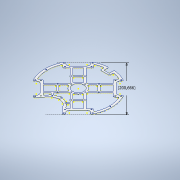
# Autodesk Inventor part: upper_plate_04
Saved by Autodesk Inventor 2020 (Build 240168000, 168)
## iProperties
Created: 2023-12-20
Part Number: upper_plate_04
Material: Алюминий 6061
Document SubType Name: Modeling
Designer: denis
Density: 2.71714 g/cm^3
Appearance: Алюминий — плоский
Mass: 51 g
Surface Area: 248.649 cm^2
Volume: 18.7698 cm^3
Author: denis
Autodesk Inventor part; units mm, degrees
(part 1 of 3)
ref_plane "YZ Plane" through (0, 0, 0) normal (1, 0, 0) x (0, 1, 0)
ref_plane "XZ Plane" through (0, 0, 0) normal (0, 1, 0) x (-1, 0, 0)
ref_plane "XY Plane" through (0, 0, 0) normal (0, 0, 1) x (1, 0, 0)
sketch "Эскиз1" plane through (0, 0, 0) normal (0, 1, 0) x (-1, 0, 0)
  arc A0 (93.0503, -48.6481) -> (93.0503, 48.6481) centre (0, 0) ccw
  line L0 (0, 0) -> (0, -105) construction
  line L1 (0, 0) -> (105, 0) construction
  line L2 (0, 0) -> (74.2462, -74.2462) construction
  line L3 (0, 0) -> (105, 0) construction
  arc A1 (47.0668, -85.9577) -> (85.9577, -47.0668) centre (0, 0) ccw construction
  line L4 (0, 0) -> (-74.2462, -74.2462) construction
  line L5 (73.8927, -46.3155) -> (46.3155, -73.8927)
  line L6 (76.014, -34.2947) -> (34.2947, -76.014)
  circle A2 centre (37.8302, -79.5495) radius 1.6
  circle A3 centre (79.5495, -37.8302) radius 1.6
  line L7 (37.8302, -79.5495) -> (79.5495, -37.8302) construction
  line L8 (87.1795, -38.3892) -> (83.085, -34.2947)
  line L9 (38.3892, -87.1795) -> (34.2947, -83.085)
  line L10 (88.2704, -49.3795) -> (85.2064, -46.3155)
  line L11 (49.3795, -88.2704) -> (46.3155, -85.2064)
  arc A4 (74.2462, -74.2462) -> (91.1, -52.2091) centre (0, 0) ccw construction
  arc A5 (52.2091, -91.1) -> (74.2462, -74.2462) centre (0, 0) ccw construction
  arc A6 (48.6481, -93.0503) -> (49.3795, -88.2704) centre (47.2582, -90.3917) ccw
  arc A7 (88.2704, -49.3795) -> (93.0503, -48.6481) centre (90.3917, -47.2582) ccw
  arc A8 (46.3155, -73.8927) -> (46.3155, -85.2064) centre (51.9723, -79.5495) ccw
  arc A9 (85.2064, -46.3155) -> (73.8927, -46.3155) centre (79.5495, -51.9723) ccw
  arc A10 (34.2947, -76.014) -> (34.2947, -83.085) centre (37.8302, -79.5495) ccw
  arc A11 (83.085, -34.2947) -> (76.014, -34.2947) centre (79.5495, -37.8302) ccw
  arc A12 (40.4652, -89.2556) -> (47.0668, -85.9577) centre (0, 0) ccw construction
  arc A13 (85.9577, -47.0668) -> (89.2556, -40.4652) centre (0, 0) ccw construction
  arc A14 (90.4395, -37.7453) -> (90.4395, 37.7453) centre (0, 0) ccw
  arc A15 (87.1795, -38.3892) -> (90.4395, -37.7453) centre (88.5938, -36.975) ccw
  arc A16 (37.7453, -90.4395) -> (38.3892, -87.1795) centre (36.975, -88.5938) ccw
  arc A17 (38.3892, 87.1795) -> (37.7453, 90.4395) centre (36.975, 88.5938) ccw construction
  arc A18 (49.3795, 88.2704) -> (48.6481, 93.0503) centre (47.2582, 90.3917) ccw
  line L12 (49.3795, 88.2704) -> (46.3155, 85.2064)
  arc A19 (46.3155, 85.2064) -> (46.3155, 73.8927) centre (51.9723, 79.5495) ccw
  line L13 (38.3892, 87.1795) -> (34.2947, 83.085) construction
  arc A20 (34.2947, 83.085) -> (34.2947, 76.014) centre (37.8302, 79.5495) ccw construction
  line L14 (34.2947, 76.014) -> (76.014, 34.2947) construction
  line L15 (46.3155, 73.8927) -> (73.8927, 46.3155)
  arc A21 (76.014, 34.2947) -> (83.085, 34.2947) centre (79.5495, 37.8302) ccw
  circle A22 centre (37.8302, 79.5495) radius 1.6
  circle A23 centre (79.5495, 37.8302) radius 1.6
  line L16 (87.1795, 38.3892) -> (83.085, 34.2947)
  arc A24 (90.4395, 37.7453) -> (87.1795, 38.3892) centre (88.5938, 36.975) ccw
  arc A25 (93.0503, 48.6481) -> (88.2704, 49.3795) centre (90.3917, 47.2582) ccw
  line L17 (88.2704, 49.3795) -> (85.2064, 46.3155)
  arc A26 (73.8927, 46.3155) -> (85.2064, 46.3155) centre (79.5495, 51.9723) ccw
  arc A27 (-87.1795, 38.3892) -> (-90.4395, 37.7453) centre (-88.5938, 36.975) ccw
  arc A28 (-88.2704, 49.3795) -> (-93.0503, 48.6481) centre (-90.3917, 47.2582) ccw
  line L18 (-88.2704, 49.3795) -> (-85.2064, 46.3155)
  arc A29 (-85.2064, 46.3155) -> (-73.8927, 46.3155) centre (-79.5495, 51.9723) ccw
  line L19 (-87.1795, 38.3892) -> (-83.085, 34.2947)
  arc A30 (-83.085, 34.2947) -> (-76.014, 34.2947) centre (-79.5495, 37.8302) ccw
  line L20 (-76.014, 34.2947) -> (-34.2947, 76.014) construction
  line L21 (-73.8927, 46.3155) -> (-46.3155, 73.8927)
  arc A31 (-34.2947, 76.014) -> (-34.2947, 83.085) centre (-37.8302, 79.5495) ccw construction
  circle A32 centre (-79.5495, 37.8302) radius 1.6
  circle A33 centre (-37.8302, 79.5495) radius 1.6
  line L22 (-38.3892, 87.1795) -> (-34.2947, 83.085) construction
  arc A34 (-37.7453, 90.4395) -> (-38.3892, 87.1795) centre (-36.975, 88.5938) ccw construction
  arc A35 (-48.6481, 93.0503) -> (-49.3795, 88.2704) centre (-47.2582, 90.3917) ccw
  line L23 (-49.3795, 88.2704) -> (-46.3155, 85.2064)
  arc A36 (-46.3155, 73.8927) -> (-46.3155, 85.2064) centre (-51.9723, 79.5495) ccw
  arc A37 (-38.3892, -87.1795) -> (-37.7453, -90.4395) centre (-36.975, -88.5938) ccw
  arc A38 (-49.3795, -88.2704) -> (-48.6481, -93.0503) centre (-47.2582, -90.3917) ccw
  line L24 (-49.3795, -88.2704) -> (-46.3155, -85.2064)
  arc A39 (-46.3155, -85.2064) -> (-46.3155, -73.8927) centre (-51.9723, -79.5495) ccw
  line L25 (-38.3892, -87.1795) -> (-34.2947, -83.085)
  arc A40 (-34.2947, -83.085) -> (-34.2947, -76.014) centre (-37.8302, -79.5495) ccw
  line L26 (-34.2947, -76.014) -> (-76.014, -34.2947)
  line L27 (-46.3155, -73.8927) -> (-73.8927, -46.3155)
  arc A41 (-76.014, -34.2947) -> (-83.085, -34.2947) centre (-79.5495, -37.8302) ccw
  circle A42 centre (-37.8302, -79.5495) radius 1.6
  circle A43 centre (-79.5495, -37.8302) radius 1.6
  line L28 (-87.1795, -38.3892) -> (-83.085, -34.2947)
  arc A44 (-90.4395, -37.7453) -> (-87.1795, -38.3892) centre (-88.5938, -36.975) ccw
  arc A45 (-93.0503, -48.6481) -> (-88.2704, -49.3795) centre (-90.3917, -47.2582) ccw
  line L29 (-88.2704, -49.3795) -> (-85.2064, -46.3155)
  arc A46 (-73.8927, -46.3155) -> (-85.2064, -46.3155) centre (-79.5495, -51.9723) ccw
  arc A47 (0, 67.941) -> (23.7825, 76.5969) centre (0, 104.941) ccw construction
  arc A48 (-23.7825, 76.5969) -> (0, 67.941) centre (0, 104.941) ccw construction
  line L30 (-23.7825, 76.5969) -> (-29.1816, 81.127) construction
  arc A49 (-28.5452, 71.4571) -> (5.5413, 61.2914) centre (0, 104.941) ccw construction
  arc A50 (5.5413, 61.2914) -> (28.5452, 71.4571) centre (0, 104.941) ccw construction
  line L31 (23.7825, 76.5969) -> (26.8032, 79.1314) construction
  line L32 (-34.1491, 76.1596) -> (-28.5452, 71.4571) construction
  line L33 (31.2232, 73.7044) -> (28.5452, 71.4571) construction
  line L34 (26.8032, 79.1314) -> (23.7825, 76.5969) construction
  line L35 (30.7591, 79.5495) -> (31.4483, 78.8604) construction
  line L36 (31.2232, 73.7044) -> (28.5452, 71.4571) construction
  line L37 (-28.5452, 71.4571) -> (-34.1491, 76.1596) construction
  line L38 (-23.7825, 76.5969) -> (-29.1816, 81.127) construction
  line L39 (-29.1816, 81.127) -> (-34.1491, 76.1596) construction
  arc A51 (31.2232, 73.7044) -> (26.6462, 78.9996) centre (28.9734, 76.3855) ccw construction
  arc A52 (-26.6462, 78.9996) -> (-31.2232, 73.7044) centre (-28.9734, 76.3855) ccw construction
  arc A53 (-24.842, 61.8893) -> (-25.4187, 62.8242) centre (-28.1154, 60.5155) ccw
  line L40 (-24.842, 61.8893) -> (-23.8313, 59.4808)
  line L41 (-43.0355, 94.1655) -> (-18.3802, 65.3664)
  arc A54 (-0.6161, 59.3045) -> (0.6161, 59.3045) centre (0, 61.2072) ccw
  line L42 (-2.672, 59.9702) -> (-4.5, 60.5621) construction
  arc A55 (-2.5156, 60.0805) -> (-2.672, 59.9702) centre (0, 56.3493) ccw construction
  line L43 (-15.1585, 56.5907) -> (-21.0049, 57.3328)
  arc A56 (-14.5119, 56.4463) -> (-15.1585, 56.5907) centre (-15.6055, 53.069) ccw
  line L44 (-17.477, 64.7643) -> (-0.6161, 59.3045)
  line L45 (-14.5119, 56.4463) -> (-0.6161, 51.9466)
  arc A57 (44.0271, 95.3237) -> (43.577, 95.5303) centre (0, 0) ccw construction
  circle A58 centre (20.5578, 60.8546) radius 1.55
  arc A59 (-34.1909, 73.0707) -> (-37.1244, 73.1843) centre (-35.7102, 71.7701) ccw
  line L46 (-34.1909, 73.0707) -> (-27.0558, 64.7365) construction
  line L47 (-25.4187, 62.8242) -> (-34.1909, 73.0707)
  arc A60 (-23.8313, 59.4808) -> (-21.0049, 57.3328) centre (-20.5578, 60.8546) ccw
  arc A61 (-18.3802, 65.3664) -> (-17.477, 64.7643) centre (-16.8609, 66.6671) ccw
  circle A62 centre (-20.5578, 60.8546) radius 1.55
  arc A63 (15.1585, 56.5907) -> (14.5119, 56.4463) centre (15.6055, 53.069) ccw
  line L48 (15.1585, 56.5907) -> (21.0049, 57.3328)
  arc A64 (25.4187, 62.8242) -> (24.842, 61.8893) centre (28.1154, 60.5155) ccw
  line L49 (24.842, 61.8893) -> (23.8313, 59.4808)
  arc A65 (21.0049, 57.3328) -> (23.8313, 59.4808) centre (20.5578, 60.8546) ccw
  line L50 (25.4187, 62.8242) -> (34.1909, 73.0707)
  arc A66 (37.1244, 73.1843) -> (34.1909, 73.0707) centre (35.7102, 71.7701) ccw
  line L51 (14.5119, 56.4463) -> (0.6161, 51.9466)
  arc A67 (17.477, 64.7643) -> (18.3802, 65.3664) centre (16.8609, 66.6671) ccw
  line L52 (17.477, 64.7643) -> (0.6161, 59.3045)
  line L53 (-37.1244, 73.1843) -> (-76.014, 34.2947)
  line L54 (37.1244, 73.1843) -> (76.014, 34.2947)
  arc A68 (-45.42, 94.668) -> (-48.6481, 93.0503) centre (0, 0) ccw
  arc A69 (-43.0355, 94.1655) -> (-45.42, 94.668) centre (-44.5548, 92.8648) ccw
  arc A70 (-0.6161, 51.9466) -> (0.6161, 51.9466) centre (0, 53.8493) ccw
  arc A71 (-48.6481, 93.0503) -> (-93.0503, 48.6481) centre (0, 0) ccw construction
  line L55 (43.0355, 94.1655) -> (18.3802, 65.3664)
  arc A72 (48.6481, 93.0503) -> (45.42, 94.668) centre (0, 0) ccw
  arc A73 (45.42, 94.668) -> (43.0355, 94.1655) centre (44.5548, 92.8648) ccw
  arc A74 (93.0503, 48.6481) -> (-44.0271, 95.3237) centre (0, 0) ccw construction
  arc A75 (-93.0503, -48.6481) -> (-48.6481, -93.0503) centre (0, 0) ccw construction
  arc A76 (-93.0503, 48.6481) -> (-93.0503, -48.6481) centre (0, 0) ccw
  arc A77 (-90.4395, -37.7453) -> (-37.7453, -90.4395) centre (0, 0) ccw construction
  arc A78 (-90.4395, 37.7453) -> (-90.4395, -37.7453) centre (0, 0) ccw
  arc A79 (90.4395, 37.7453) -> (-90.4395, 37.7453) centre (0, 0) ccw construction
  arc A80 (-37.7453, -90.4395) -> (37.7453, -90.4395) centre (0, 0) ccw
  arc A81 (-48.6481, -93.0503) -> (48.6481, -93.0503) centre (0, 0) ccw
  circle A82 centre (0, 55.4493) radius 1.6
  point P0 (60.1041, -60.1041)
  point P1 (55.1543, -55.1543)
  point P2 (78.1353, -39.2444)
  point P3 (39.2444, -78.1353)
  point P4 (52.2091, 91.1)
  point P5 (39.2444, 78.1353)
  point P6 (47.0668, 85.9577)
  point P7 (55.1543, 55.1543)
  point P8 (60.1041, 60.1041)
  point P9 (91.1, 52.2091)
  point P10 (78.1353, 39.2444)
  point P11 (85.9577, 47.0668)
  point P12 (-91.1, 52.2091)
  point P13 (-78.1353, 39.2444)
  point P14 (-85.9577, 47.0668)
  point P15 (-55.1543, 55.1543)
  point P16 (-60.1041, 60.1041)
  point P17 (-52.2091, 91.1)
  point P18 (-39.2444, 78.1353)
  point P19 (-47.0668, 85.9577)
  point P20 (-52.2091, -91.1)
  point P21 (-39.2444, -78.1353)
  point P22 (-47.0668, -85.9577)
  point P23 (-55.1543, -55.1543)
  point P24 (-60.1041, -60.1041)
  point P25 (-91.1, -52.2091)
  point P26 (-78.1353, -39.2444)
  point P27 (-85.9577, -47.0668)
  point P28 (-28.5452, 71.4571)
  point P29 (-39.283, 89.7822)
  point P30 (0, 95.3237)
  point P31 (0, 66.2072)
  point P32 (-44.0271, 95.3237)
  point P33 (0, 59.2072)
  point P34 (44.5548, 92.8648)
  point P35 (-42.4264, 67.8823)
  point P36 (-22.7059, 58.0282)
  point P37 (-21.4957, 59.6205)
  dimension "d1" = 45
  dimension "d3" = 7
  dimension "d5" = 20
  dimension "d9" = 7
  dimension "d10" = 3.2
  dimension "d14" = 59
  dimension "d15" = 83
  dimension "d17" = 69
  dimension "d19" = 55
  dimension "d20" = 3
  dimension "d21" = 8
  dimension "d22" = 5
  dimension "d23" = 2
  dimension "d26" = 360
  dimension "d39" = 7
  dimension "d44" = 120
  dimension "d45" = 3.55
  dimension "d46" = 2
  dimension "d47" = 2.6119
  dimension "d48" = 2
  dimension "d49" = 105
  dimension "d50" = 2
  dimension "d54" = 3.2
  dimension "d55" = 2
  constraints: 165 point on circle, 112 end point, 83 centre point, 38 point on line, 27 tangent, 23 symmetric about line, 8 midpoint, 6 equal radius, 4 coincident, 4 collinear, 4 parallel, 3 horizontal, 2 vertical, 1 equal length, 1 perpendicular, 234 other
  measures "d1" angle of L2 L3
  measures "d3" radial gap between concentric circles of A0 A1
  measures "d5" distance from line of L5 L2.end
  measures "d9" distance between parallel lines of L5 L6
  measures "d10" diameter of A2
  measures "d14" distance of L7.end L7.start
  measures "d15" distance from line of point (0, 0) L7
  measures "d17" distance between parallel lines of L8 L9
  measures "d19" distance between parallel lines of L11 L10
  measures "d20" radius of A6
  measures "d21" radius of A8
  measures "d22" radius of A10
  measures "d23" radius of A15
  measures "d39" distance of point (0, 66.207) point (0, 59.207)
  measures "d44" angle of L40 L43
  measures "d45" radius of A53
  measures "d46" distance of point (-22.706, 58.028) point (-21.496, 59.621)
  measures "d47" distance of L40.start L40.end
  measures "d48" radius of A69
  measures "d49" radius of A68
  measures "d50" radius of A70
  measures "d54" diameter of A82
extrude "outer" add sketch "Эскиз1" along normal blind 2 contours A7 L10 A9 L5 A8 L11 A6 A81 A38 L24 A39 L27 A46 L29 A45 A76 A28 L18 A29 L21 A36 L23 A35 A68 A69 L41 A61 L44 A54 L52 A67 L55 A73 A72 A18 L12 A19 L15 A26 L17 A25 A0 | A82
sketch "Эскиз2" plane through (0, 2, 0) normal (0, 1, 0) x (1, 0, 0)
  circle A0 centre (0, 0) radius 18
  arc A1 (-16.2635, 16.2635) -> (-21.4111, 8.4003) centre (0, 0) ccw
  line L0 (0, 0) -> (-74.2462, 74.2462) construction
  line L1 (0, 0) -> (-105, 0) construction
  line L2 (0, 0) -> (0, 105) construction
  line L3 (0, 0) -> (74.2462, 74.2462) construction
  line L4 (-46.669, 63.6396) -> (-27.2236, 44.1942)
  line L5 (-63.6396, 46.669) -> (-44.1942, 27.2236)
  arc A2 (-46.3155, -85.2064) -> (-46.3155, -73.8927) centre (-51.9723, -79.5495) ccw construction
  line L6 (-46.3155, -85.2064) -> (-49.3795, -88.2704) construction
  arc A3 (-49.3795, -88.2704) -> (-48.6481, -93.0503) centre (-47.2582, -90.3917) ccw construction
  arc A4 (-48.6481, -93.0503) -> (-45.42, -94.668) centre (0, 0) ccw construction
  arc A5 (-45.42, -94.668) -> (-43.0355, -94.1655) centre (-44.5548, -92.8648) ccw construction
  line L7 (-43.0355, -94.1655) -> (-18.3802, -65.3664) construction
  arc A6 (-17.477, -64.7643) -> (-18.3802, -65.3664) centre (-16.8609, -66.6671) ccw construction
  line L8 (-17.477, -64.7643) -> (-0.6161, -59.3045) construction
  arc A7 (0.6161, -59.3045) -> (-0.6161, -59.3045) centre (0, -61.2072) ccw construction
  line L9 (0.6161, -59.3045) -> (17.477, -64.7643) construction
  arc A8 (18.3802, -65.3664) -> (17.477, -64.7643) centre (16.8609, -66.6671) ccw construction
  line L10 (18.3802, -65.3664) -> (43.0355, -94.1655) construction
  arc A9 (43.0355, -94.1655) -> (45.42, -94.668) centre (44.5548, -92.8648) ccw construction
  arc A10 (45.42, -94.668) -> (48.6481, -93.0503) centre (0, 0) ccw construction
  arc A11 (48.6481, -93.0503) -> (49.3795, -88.2704) centre (47.2582, -90.3917) ccw construction
  line L11 (49.3795, -88.2704) -> (46.3155, -85.2064) construction
  arc A12 (46.3155, -73.8927) -> (46.3155, -85.2064) centre (51.9723, -79.5495) ccw construction
  line L12 (46.3155, -73.8927) -> (73.8927, -46.3155) construction
  arc A13 (85.2064, -46.3155) -> (73.8927, -46.3155) centre (79.5495, -51.9723) ccw construction
  line L13 (85.2064, -46.3155) -> (88.2704, -49.3795) construction
  arc A14 (88.2704, -49.3795) -> (93.0503, -48.6481) centre (90.3917, -47.2582) ccw construction
  arc A15 (93.0503, -48.6481) -> (93.0503, 48.6481) centre (0, 0) ccw construction
  arc A16 (93.0503, 48.6481) -> (88.2704, 49.3795) centre (90.3917, 47.2582) ccw construction
  line L14 (88.2704, 49.3795) -> (85.2064, 46.3155) construction
  arc A17 (73.8927, 46.3155) -> (85.2064, 46.3155) centre (79.5495, 51.9723) ccw construction
  line L15 (73.8927, 46.3155) -> (46.3155, 73.8927) construction
  arc A18 (46.3155, 85.2064) -> (46.3155, 73.8927) centre (51.9723, 79.5495) ccw construction
  line L16 (46.3155, 85.2064) -> (49.3795, 88.2704) construction
  arc A19 (49.3795, 88.2704) -> (48.6481, 93.0503) centre (47.2582, 90.3917) ccw construction
  arc A20 (48.6481, 93.0503) -> (-48.6481, 93.0503) centre (0, 0) ccw construction
  arc A21 (-48.6481, 93.0503) -> (-49.3795, 88.2704) centre (-47.2582, 90.3917) ccw construction
  line L17 (-49.3795, 88.2704) -> (-46.3155, 85.2064) construction
  arc A22 (-46.3155, 73.8927) -> (-46.3155, 85.2064) centre (-51.9723, 79.5495) ccw construction
  line L18 (-46.3155, 73.8927) -> (-73.8927, 46.3155) construction
  arc A23 (-85.2064, 46.3155) -> (-73.8927, 46.3155) centre (-79.5495, 51.9723) ccw construction
  line L19 (-85.2064, 46.3155) -> (-88.2704, 49.3795) construction
  arc A24 (-88.2704, 49.3795) -> (-93.0503, 48.6481) centre (-90.3917, 47.2582) ccw construction
  arc A25 (-93.0503, 48.6481) -> (-93.0503, -48.6481) centre (0, 0) ccw construction
  arc A26 (-93.0503, -48.6481) -> (-88.2704, -49.3795) centre (-90.3917, -47.2582) ccw construction
  line L20 (-88.2704, -49.3795) -> (-85.2064, -46.3155) construction
  arc A27 (-73.8927, -46.3155) -> (-85.2064, -46.3155) centre (-79.5495, -51.9723) ccw construction
  line L21 (-73.8927, -46.3155) -> (-46.3155, -73.8927) construction
  circle A28 centre (-37.8302, 79.5495) radius 1.6 construction
  circle A29 centre (-79.5495, 37.8302) radius 1.6 construction
  circle A30 centre (-79.5495, -37.8302) radius 1.6 construction
  circle A31 centre (79.5495, -37.8302) radius 1.6 construction
  circle A32 centre (37.8302, 79.5495) radius 1.6 construction
  circle A33 centre (79.5495, 37.8302) radius 1.6 construction
  circle A34 centre (-20.5578, -60.8546) radius 1.55 construction
  circle A35 centre (20.5578, -60.8546) radius 1.55 construction
  circle A36 centre (37.8302, -79.5495) radius 1.6 construction
  circle A37 centre (-37.8302, -79.5495) radius 1.6 construction
  line L22 (-83.085, -34.2947) -> (-87.1795, -38.3892) construction
  arc A38 (-90.4395, -37.7453) -> (-87.1795, -38.3892) centre (-88.5938, -36.975) ccw construction
  arc A39 (-90.4395, 37.7453) -> (-90.4395, -37.7453) centre (0, 0) ccw construction
  arc A40 (-87.1795, 38.3892) -> (-90.4395, 37.7453) centre (-88.5938, 36.975) ccw construction
  line L23 (-87.1795, 38.3892) -> (-83.085, 34.2947) construction
  arc A41 (-83.085, 34.2947) -> (-76.014, 34.2947) centre (-79.5495, 37.8302) ccw construction
  line L24 (-76.014, 34.2947) -> (-34.2947, 76.014) projected
  arc A42 (-34.2947, 76.014) -> (-34.2947, 83.085) centre (-37.8302, 79.5495) ccw construction
  line L25 (-34.2947, 83.085) -> (-38.3892, 87.1795) construction
  arc A43 (-37.7453, 90.4395) -> (-38.3892, 87.1795) centre (-36.975, 88.5938) ccw construction
  arc A44 (37.7453, 90.4395) -> (-37.7453, 90.4395) centre (0, 0) ccw construction
  arc A45 (38.3892, 87.1795) -> (37.7453, 90.4395) centre (36.975, 88.5938) ccw construction
  line L26 (38.3892, 87.1795) -> (34.2947, 83.085) construction
  arc A46 (34.2947, 83.085) -> (34.2947, 76.014) centre (37.8302, 79.5495) ccw construction
  line L27 (34.2947, 76.014) -> (76.014, 34.2947) projected
  arc A47 (76.014, 34.2947) -> (83.085, 34.2947) centre (79.5495, 37.8302) ccw construction
  line L28 (83.085, 34.2947) -> (87.1795, 38.3892) construction
  arc A48 (90.4395, 37.7453) -> (87.1795, 38.3892) centre (88.5938, 36.975) ccw construction
  arc A49 (90.4395, -37.7453) -> (90.4395, 37.7453) centre (0, 0) ccw construction
  arc A50 (87.1795, -38.3892) -> (90.4395, -37.7453) centre (88.5938, -36.975) ccw construction
  line L29 (87.1795, -38.3892) -> (83.085, -34.2947) construction
  arc A51 (83.085, -34.2947) -> (76.014, -34.2947) centre (79.5495, -37.8302) ccw construction
  line L30 (76.014, -34.2947) -> (37.1244, -73.1843) projected
  arc A52 (34.1909, -73.0707) -> (37.1244, -73.1843) centre (35.7102, -71.7701) ccw construction
  line L31 (34.1909, -73.0707) -> (25.4187, -62.8242) construction
  arc A53 (24.842, -61.8893) -> (25.4187, -62.8242) centre (28.1154, -60.5155) ccw construction
  line L32 (24.842, -61.8893) -> (23.8313, -59.4808) construction
  arc A54 (23.8313, -59.4808) -> (21.0049, -57.3328) centre (20.5578, -60.8546) ccw construction
  line L33 (21.0049, -57.3328) -> (15.1585, -56.5907) construction
  arc A55 (14.5119, -56.4463) -> (15.1585, -56.5907) centre (15.6055, -53.069) ccw construction
  line L34 (14.5119, -56.4463) -> (0.6161, -51.9466) construction
  arc A56 (0.6161, -51.9466) -> (-0.6161, -51.9466) centre (0, -53.8493) ccw construction
  line L35 (-0.6161, -51.9466) -> (-14.5119, -56.4463) construction
  arc A57 (-15.1585, -56.5907) -> (-14.5119, -56.4463) centre (-15.6055, -53.069) ccw construction
  line L36 (-15.1585, -56.5907) -> (-21.0049, -57.3328) construction
  arc A58 (-21.0049, -57.3328) -> (-23.8313, -59.4808) centre (-20.5578, -60.8546) ccw construction
  line L37 (-23.8313, -59.4808) -> (-24.842, -61.8893) construction
  arc A59 (-25.4187, -62.8242) -> (-24.842, -61.8893) centre (-28.1154, -60.5155) ccw construction
  line L38 (-25.4187, -62.8242) -> (-34.1909, -73.0707) construction
  arc A60 (-37.1244, -73.1843) -> (-34.1909, -73.0707) centre (-35.7102, -71.7701) ccw construction
  line L39 (-37.1244, -73.1843) -> (-76.014, -34.2947) projected
  arc A61 (-76.014, -34.2947) -> (-83.085, -34.2947) centre (-79.5495, -37.8302) ccw construction
  line L40 (-42.4264, 67.8823) -> (-1.4142, 26.8701)
  line L41 (-41.3657, 27.2236) -> (-27.2236, 41.3657)
  line L42 (-37.8302, 23.6881) -> (-23.6881, 37.8302)
  circle A62 centre (-21.9203, 43.1335) radius 1.6
  circle A63 centre (-43.1335, 21.9203) radius 1.6
  line L43 (-43.1335, 21.9203) -> (-21.9203, 43.1335) construction
  arc A64 (-27.2236, 41.3657) -> (-27.2236, 44.1942) centre (-28.6378, 42.78) ccw
  arc A65 (-44.1942, 27.2236) -> (-41.3657, 27.2236) centre (-42.78, 28.6378) ccw
  line L44 (-20.8597, 37.8302) -> (-7.7166, 24.6871)
  line L45 (-37.8302, 20.8597) -> (-24.6871, 7.7166)
  arc A66 (-20.8597, 37.8302) -> (-23.6881, 37.8302) centre (-22.2739, 36.416) ccw
  arc A67 (-37.8302, 23.6881) -> (-37.8302, 20.8597) centre (-36.416, 22.2739) ccw
  line L46 (42.4264, 67.8823) -> (1.4142, 26.8701) construction
  arc A68 (-1.4142, 26.8701) -> (1.4142, 26.8701) centre (0, 28.2843) ccw
  arc A69 (-8.4003, 21.4111) -> (-16.2635, 16.2635) centre (0, 0) ccw
  arc A70 (-22.3597, 5.3892) -> (-5.3892, 22.3597) centre (0, 0) ccw construction
  arc A71 (-8.4003, 21.4111) -> (-7.7166, 24.6871) centre (-9.1308, 23.2729) ccw
  arc A72 (-24.6871, 7.7166) -> (-21.4111, 8.4003) centre (-23.2729, 9.1308) ccw
  line L47 (-67.8823, 42.4264) -> (-42.4264, 67.8823) construction
  line L48 (-67.8823, 42.4264) -> (-26.8701, 1.4142)
  line L49 (-67.8823, -42.4264) -> (-26.8701, -1.4142)
  line L50 (-42.4264, -67.8823) -> (-1.4142, -26.8701)
  line L51 (-46.669, -63.6396) -> (-27.2236, -44.1942)
  arc A73 (-27.2236, -44.1942) -> (-27.2236, -41.3657) centre (-28.6378, -42.78) ccw
  line L52 (-27.2236, -41.3657) -> (-41.3657, -27.2236)
  arc A74 (-41.3657, -27.2236) -> (-44.1942, -27.2236) centre (-42.78, -28.6378) ccw
  line L53 (-63.6396, -46.669) -> (-44.1942, -27.2236)
  line L54 (-37.8302, -20.8597) -> (-24.6871, -7.7166)
  line L55 (-23.6881, -37.8302) -> (-37.8302, -23.6881)
  arc A75 (-21.4111, -8.4003) -> (-16.2635, -16.2635) centre (0, 0) ccw
  arc A76 (-16.2635, -16.2635) -> (-8.4003, -21.4111) centre (0, 0) ccw
  arc A77 (-7.7166, -24.6871) -> (-8.4003, -21.4111) centre (-9.1308, -23.2729) ccw
  line L56 (-20.8597, -37.8302) -> (-7.7166, -24.6871)
  arc A78 (-23.6881, -37.8302) -> (-20.8597, -37.8302) centre (-22.2739, -36.416) ccw
  arc A79 (-37.8302, -20.8597) -> (-37.8302, -23.6881) centre (-36.416, -22.2739) ccw
  arc A80 (-21.4111, -8.4003) -> (-24.6871, -7.7166) centre (-23.2729, -9.1308) ccw
  circle A81 centre (-21.9203, -43.1335) radius 1.6
  circle A82 centre (-43.1335, -21.9203) radius 1.6
  arc A83 (-26.8701, -1.4142) -> (-26.8701, 1.4142) centre (-28.2843, 0) ccw
  line L57 (42.4264, -67.8823) -> (1.4142, -26.8701)
  line L58 (67.8823, -42.4264) -> (26.8701, -1.4142)
  line L59 (63.6396, -46.669) -> (44.1942, -27.2236)
  arc A84 (44.1942, -27.2236) -> (41.3657, -27.2236) centre (42.78, -28.6378) ccw
  line L60 (41.3657, -27.2236) -> (27.2236, -41.3657)
  arc A85 (27.2236, -41.3657) -> (27.2236, -44.1942) centre (28.6378, -42.78) ccw
  line L61 (46.669, -63.6396) -> (27.2236, -44.1942)
  line L62 (20.8597, -37.8302) -> (7.7166, -24.6871)
  line L63 (37.8302, -23.6881) -> (23.6881, -37.8302)
  arc A86 (8.4003, -21.4111) -> (16.2635, -16.2635) centre (0, 0) ccw
  arc A87 (16.2635, -16.2635) -> (21.4111, -8.4003) centre (0, 0) ccw
  arc A88 (24.6871, -7.7166) -> (21.4111, -8.4003) centre (23.2729, -9.1308) ccw
  line L64 (37.8302, -20.8597) -> (24.6871, -7.7166)
  arc A89 (37.8302, -23.6881) -> (37.8302, -20.8597) centre (36.416, -22.2739) ccw
  arc A90 (20.8597, -37.8302) -> (23.6881, -37.8302) centre (22.2739, -36.416) ccw
  arc A91 (8.4003, -21.4111) -> (7.7166, -24.6871) centre (9.1308, -23.2729) ccw
  circle A92 centre (43.1335, -21.9203) radius 1.6
  circle A93 centre (21.9203, -43.1335) radius 1.6
  arc A94 (1.4142, -26.8701) -> (-1.4142, -26.8701) centre (0, -28.2843) ccw
  line L65 (67.8823, 42.4264) -> (26.8701, 1.4142)
  line L66 (42.4264, 67.8823) -> (1.4142, 26.8701)
  line L67 (46.669, 63.6396) -> (27.2236, 44.1942)
  arc A95 (27.2236, 44.1942) -> (27.2236, 41.3657) centre (28.6378, 42.78) ccw
  line L68 (27.2236, 41.3657) -> (41.3657, 27.2236)
  arc A96 (41.3657, 27.2236) -> (44.1942, 27.2236) centre (42.78, 28.6378) ccw
  line L69 (63.6396, 46.669) -> (44.1942, 27.2236)
  line L70 (37.8302, 20.8597) -> (24.6871, 7.7166)
  line L71 (23.6881, 37.8302) -> (37.8302, 23.6881)
  arc A97 (21.4111, 8.4003) -> (16.2635, 16.2635) centre (0, 0) ccw
  arc A98 (16.2635, 16.2635) -> (8.4003, 21.4111) centre (0, 0) ccw
  arc A99 (7.7166, 24.6871) -> (8.4003, 21.4111) centre (9.1308, 23.2729) ccw
  line L72 (20.8597, 37.8302) -> (7.7166, 24.6871)
  arc A100 (23.6881, 37.8302) -> (20.8597, 37.8302) centre (22.2739, 36.416) ccw
  arc A101 (37.8302, 20.8597) -> (37.8302, 23.6881) centre (36.416, 22.2739) ccw
  arc A102 (21.4111, 8.4003) -> (24.6871, 7.7166) centre (23.2729, 9.1308) ccw
  circle A103 centre (21.9203, 43.1335) radius 1.6
  circle A104 centre (43.1335, 21.9203) radius 1.6
  arc A105 (26.8701, 1.4142) -> (26.8701, -1.4142) centre (28.2843, 0) ccw
  circle A106 centre (0, 0) radius 22 construction
  circle A107 centre (0, 22) radius 1.6
  circle A108 centre (-22, 0) radius 1.6
  circle A109 centre (0, -22) radius 1.6
  circle A110 centre (22, 0) radius 1.6
  circle A111 centre (21.9203, -43.1335) radius 4
  circle A112 centre (43.1335, -21.9203) radius 4
  circle A113 centre (-21.9203, -43.1335) radius 4
  circle A114 centre (-43.1335, -21.9203) radius 4
  circle A115 centre (21.9203, 43.1335) radius 4
  circle A116 centre (43.1335, 21.9203) radius 4
  circle A117 centre (-21.9203, 43.1335) radius 4
  circle A118 centre (-43.1335, 21.9203) radius 4
  point P0 (0, 25.4558)
  point P1 (-5.3892, 22.3597)
  point P2 (-22.3597, 5.3892)
  point P3 (-39.2444, 22.2739)
  point P4 (-22.2739, 39.2444)
  point P5 (-22.2739, 39.2444)
  point P6 (-39.2444, 22.2739)
  point P7 (-25.4558, 0)
  point P8 (-22.2739, -39.2444)
  point P9 (-5.3892, -22.3597)
  point P10 (-39.2444, -22.2739)
  point P11 (-22.3597, -5.3892)
  point P12 (-39.2444, -22.2739)
  point P13 (-22.2739, -39.2444)
  point P14 (0, -25.4558)
  point P15 (39.2444, -22.2739)
  point P16 (22.3597, -5.3892)
  point P17 (22.2739, -39.2444)
  point P18 (5.3892, -22.3597)
  point P19 (22.2739, -39.2444)
  point P20 (39.2444, -22.2739)
  point P21 (25.4558, 0)
  point P22 (22.2739, 39.2444)
  point P23 (5.3892, 22.3597)
  point P24 (39.2444, 22.2739)
  point P25 (22.3597, 5.3892)
  point P26 (39.2444, 22.2739)
  point P27 (22.2739, 39.2444)
  point P28 (26.8701, -1.4142)
  point P29 (1.4142, 26.8701)
  point P30 (-26.8701, 1.4142)
  point P31 (-1.4142, -26.8701)
  point P32 (43.384, 17.9282)
  point P33 (47.1257, 21.6698)
  point P34 (17.9282, 43.384)
  point P35 (21.6698, 47.1257)
  point P36 (-17.9282, 43.384)
  point P37 (-21.6698, 47.1257)
  point P38 (-43.384, 17.9282)
  point P39 (-47.1257, 21.6698)
  point P40 (-43.384, -17.9282)
  point P41 (-47.1257, -21.6698)
  point P42 (-17.9282, -43.384)
  point P43 (-21.6698, -47.1257)
  point P44 (17.9282, -43.384)
  point P45 (21.6698, -47.1257)
  point P46 (43.384, -17.9282)
  point P47 (47.1257, -21.6698)
  dimension "d75" = 44
  dimension "d56" = 36
  dimension "d57" = 5
  dimension "d59" = 12
  dimension "d61" = 6
  dimension "d63" = 5
  dimension "d64" = 3.2
  dimension "d65" = 30
  dimension "d66" = 32
  dimension "d67" = 2
  dimension "d68" = 2
  dimension "d69" = 2
  dimension "d70" = 2
  dimension "d73" = 360
  dimension "d76" = 3.2
  dimension "d79" = 360
  dimension "d97" = 8
  dimension "d98" = 8
  constraints: 86 point on circle, 70 end point, 58 centre point, 50 point on line, 14 tangent, 9 symmetric about line, 5 coincident, 3 equal radius, 3 parallel, 2 perpendicular, 1 collinear, 1 vertical alignment, 246 other
  measures "d56" diameter of A0
  measures "d57" radial gap between concentric circles of A0 A1
  measures "d59" distance between parallel lines of L4 L0
  measures "d61" distance between parallel lines of L40 L4
  measures "d63" distance between parallel lines of L41 L42
  measures "d64" diameter of A62
  measures "d65" distance of L43.start L43.end
  measures "d66" distance from line of L24 L43.end
  measures "d67" radius of A64
  measures "d68" radius of A66
  measures "d69" radius of A68
  measures "d70" radius of A71
  measures "d76" diameter of A107
  measures "d97" diameter of A111
  measures "d98" diameter of A112
extrude "inner" add sketch "Эскиз2" against normal blind 2 contours L24 L40 A117 A68 L66 A115 L27 L67 A95 L68 A96 L69 L65 A116 A105 L58 A112 L30 L59 A84 L60 A85 L61 L57 A111 A94 L50 A113 L39 L51 A73 L52 A74 L53 L49 A114 A83 L48 A118 L5 A65 L41 A64 L4 | A117 L40 | L40 A117 | A118 L48 | L48 A118 | A115 L66 | L66 A115 | A114 L49 | L49 A114 | A116 L65 | L65 A116 | A113 L50 | L50 A113 | A112 L58 | L58 A112 | A111 L57 | L57 A111
sketch "Эскиз3" plane through (0, 2, 0) normal (0, 1, 0) x (1, 0, 0)
  line L0 (-67.8823, -42.4264) -> (-76.014, -34.2947) construction
  arc A0 (-76.014, -34.2947) -> (-83.085, -34.2947) centre (-79.5495, -37.8302) ccw construction
  line L1 (-83.085, -34.2947) -> (-87.1795, -38.3892) construction
  arc A1 (-90.4395, -37.7453) -> (-87.1795, -38.3892) centre (-88.5938, -36.975) ccw construction
  arc A2 (-90.4395, 37.7453) -> (-90.4395, -37.7453) centre (0, 0) ccw construction
  arc A3 (-87.1795, 38.3892) -> (-90.4395, 37.7453) centre (-88.5938, 36.975) ccw construction
  line L2 (-87.1795, 38.3892) -> (-83.085, 34.2947) construction
  arc A4 (-83.085, 34.2947) -> (-76.014, 34.2947) centre (-79.5495, 37.8302) ccw construction
  line L3 (-76.014, 34.2947) -> (-67.8823, 42.4264) construction
  line L4 (-43.384, 17.9282) -> (-26.8701, 1.4142) construction
  arc A5 (-26.8701, -1.4142) -> (-26.8701, 1.4142) centre (-28.2843, 0) ccw construction
  line L5 (-47.1257, -21.6698) -> (-67.8823, -42.4264) construction
  line L6 (-63.6396, -46.669) -> (-44.1942, -27.2236) construction
  arc A6 (-41.3657, -27.2236) -> (-44.1942, -27.2236) centre (-42.78, -28.6378) ccw construction
  line L7 (-41.3657, -27.2236) -> (-27.2236, -41.3657) construction
  arc A7 (-27.2236, -44.1942) -> (-27.2236, -41.3657) centre (-28.6378, -42.78) ccw construction
  line L8 (-27.2236, -44.1942) -> (-46.669, -63.6396) construction
  line L9 (-46.669, -63.6396) -> (-63.6396, -46.669) construction
  line L10 (-17.9282, -43.384) -> (-1.4142, -26.8701) construction
  arc A8 (1.4142, -26.8701) -> (-1.4142, -26.8701) centre (0, -28.2843) ccw construction
  line L11 (21.6698, -47.1257) -> (42.4264, -67.8823) construction
  line L12 (42.4264, -67.8823) -> (37.1244, -73.1843) construction
  arc A9 (34.1909, -73.0707) -> (37.1244, -73.1843) centre (35.7102, -71.7701) ccw construction
  line L13 (34.1909, -73.0707) -> (25.4187, -62.8242) construction
  arc A10 (24.842, -61.8893) -> (25.4187, -62.8242) centre (28.1154, -60.5155) ccw construction
  line L14 (24.842, -61.8893) -> (23.8313, -59.4808) construction
  arc A11 (23.8313, -59.4808) -> (21.0049, -57.3328) centre (20.5578, -60.8546) ccw construction
  line L15 (21.0049, -57.3328) -> (15.1585, -56.5907) construction
  arc A12 (14.5119, -56.4463) -> (15.1585, -56.5907) centre (15.6055, -53.069) ccw construction
  line L16 (14.5119, -56.4463) -> (0.6161, -51.9466) construction
  arc A13 (0.6161, -51.9466) -> (-0.6161, -51.9466) centre (0, -53.8493) ccw construction
  line L17 (-0.6161, -51.9466) -> (-14.5119, -56.4463) construction
  arc A14 (-15.1585, -56.5907) -> (-14.5119, -56.4463) centre (-15.6055, -53.069) ccw construction
  line L18 (-15.1585, -56.5907) -> (-21.0049, -57.3328) construction
  arc A15 (-21.0049, -57.3328) -> (-23.8313, -59.4808) centre (-20.5578, -60.8546) ccw construction
  line L19 (-23.8313, -59.4808) -> (-24.842, -61.8893) construction
  arc A16 (-25.4187, -62.8242) -> (-24.842, -61.8893) centre (-28.1154, -60.5155) ccw construction
  line L20 (-25.4187, -62.8242) -> (-34.1909, -73.0707) construction
  arc A17 (-37.1244, -73.1843) -> (-34.1909, -73.0707) centre (-35.7102, -71.7701) ccw construction
  line L21 (-37.1244, -73.1843) -> (-42.4264, -67.8823) construction
  line L22 (46.669, -63.6396) -> (27.2236, -44.1942) construction
  arc A18 (27.2236, -41.3657) -> (27.2236, -44.1942) centre (28.6378, -42.78) ccw construction
  line L23 (27.2236, -41.3657) -> (41.3657, -27.2236) construction
  arc A19 (44.1942, -27.2236) -> (41.3657, -27.2236) centre (42.78, -28.6378) ccw construction
  line L24 (44.1942, -27.2236) -> (63.6396, -46.669) construction
  line L25 (63.6396, -46.669) -> (46.669, -63.6396) construction
  line L26 (67.8823, -42.4264) -> (47.1257, -21.6698) construction
  arc A20 (26.8701, 1.4142) -> (26.8701, -1.4142) centre (28.2843, 0) ccw construction
  line L27 (26.8701, 1.4142) -> (43.384, 17.9282) construction
  line L28 (67.8823, 42.4264) -> (76.014, 34.2947) construction
  arc A21 (76.014, 34.2947) -> (83.085, 34.2947) centre (79.5495, 37.8302) ccw construction
  line L29 (83.085, 34.2947) -> (87.1795, 38.3892) construction
  arc A22 (90.4395, 37.7453) -> (87.1795, 38.3892) centre (88.5938, 36.975) ccw construction
  arc A23 (90.4395, -37.7453) -> (90.4395, 37.7453) centre (0, 0) ccw construction
  arc A24 (87.1795, -38.3892) -> (90.4395, -37.7453) centre (88.5938, -36.975) ccw construction
  line L30 (87.1795, -38.3892) -> (83.085, -34.2947) construction
  arc A25 (83.085, -34.2947) -> (76.014, -34.2947) centre (79.5495, -37.8302) ccw construction
  line L31 (76.014, -34.2947) -> (67.8823, -42.4264) construction
  line L32 (63.6396, 46.669) -> (44.1942, 27.2236) construction
  arc A26 (41.3657, 27.2236) -> (44.1942, 27.2236) centre (42.78, 28.6378) ccw construction
  line L33 (41.3657, 27.2236) -> (27.2236, 41.3657) construction
  arc A27 (27.2236, 44.1942) -> (27.2236, 41.3657) centre (28.6378, 42.78) ccw construction
  line L34 (27.2236, 44.1942) -> (46.669, 63.6396) construction
  line L35 (46.669, 63.6396) -> (63.6396, 46.669) construction
  line L36 (42.4264, 67.8823) -> (21.6698, 47.1257) construction
  arc A28 (-1.4142, 26.8701) -> (1.4142, 26.8701) centre (0, 28.2843) ccw construction
  line L37 (-1.4142, 26.8701) -> (-17.9282, 43.384) construction
  line L38 (-42.4264, 67.8823) -> (-34.2947, 76.014) construction
  arc A29 (-34.2947, 76.014) -> (-34.2947, 83.085) centre (-37.8302, 79.5495) ccw construction
  line L39 (-34.2947, 83.085) -> (-38.3892, 87.1795) construction
  arc A30 (-37.7453, 90.4395) -> (-38.3892, 87.1795) centre (-36.975, 88.5938) ccw construction
  arc A31 (37.7453, 90.4395) -> (-37.7453, 90.4395) centre (0, 0) ccw construction
  arc A32 (38.3892, 87.1795) -> (37.7453, 90.4395) centre (36.975, 88.5938) ccw construction
  line L40 (38.3892, 87.1795) -> (34.2947, 83.085) construction
  arc A33 (34.2947, 83.085) -> (34.2947, 76.014) centre (37.8302, 79.5495) ccw construction
  line L41 (34.2947, 76.014) -> (42.4264, 67.8823) construction
  line L42 (37.8302, -23.6881) -> (23.6881, -37.8302) construction
  arc A34 (20.8597, -37.8302) -> (23.6881, -37.8302) centre (22.2739, -36.416) ccw construction
  line L43 (20.8597, -37.8302) -> (7.7166, -24.6871) construction
  arc A35 (8.4003, -21.4111) -> (7.7166, -24.6871) centre (9.1308, -23.2729) ccw construction
  arc A36 (8.4003, -21.4111) -> (21.4111, -8.4003) centre (0, 0) ccw construction
  arc A37 (24.6871, -7.7166) -> (21.4111, -8.4003) centre (23.2729, -9.1308) ccw construction
  line L44 (24.6871, -7.7166) -> (37.8302, -20.8597) construction
  arc A38 (37.8302, -23.6881) -> (37.8302, -20.8597) centre (36.416, -22.2739) ccw construction
  circle A39 centre (-21.9203, 43.1335) radius 1.6 construction
  arc A40 (-8.4003, 21.4111) -> (-21.4111, 8.4003) centre (0, 0) ccw construction
  arc A41 (-24.6871, 7.7166) -> (-21.4111, 8.4003) centre (-23.2729, 9.1308) ccw construction
  line L45 (-24.6871, 7.7166) -> (-37.8302, 20.8597) construction
  arc A42 (-37.8302, 23.6881) -> (-37.8302, 20.8597) centre (-36.416, 22.2739) ccw construction
  line L46 (-37.8302, 23.6881) -> (-23.6881, 37.8302) construction
  arc A43 (-20.8597, 37.8302) -> (-23.6881, 37.8302) centre (-22.2739, 36.416) ccw construction
  line L47 (-20.8597, 37.8302) -> (-7.7166, 24.6871) construction
  arc A44 (-8.4003, 21.4111) -> (-7.7166, 24.6871) centre (-9.1308, 23.2729) ccw construction
  arc A45 (21.4111, 8.4003) -> (8.4003, 21.4111) centre (0, 0) ccw construction
  arc A46 (7.7166, 24.6871) -> (8.4003, 21.4111) centre (9.1308, 23.2729) ccw construction
  line L48 (7.7166, 24.6871) -> (20.8597, 37.8302) construction
  arc A47 (23.6881, 37.8302) -> (20.8597, 37.8302) centre (22.2739, 36.416) ccw construction
  line L49 (23.6881, 37.8302) -> (37.8302, 23.6881) construction
  arc A48 (37.8302, 20.8597) -> (37.8302, 23.6881) centre (36.416, 22.2739) ccw construction
  line L50 (37.8302, 20.8597) -> (24.6871, 7.7166) construction
  arc A49 (21.4111, 8.4003) -> (24.6871, 7.7166) centre (23.2729, 9.1308) ccw construction
  circle A50 centre (21.9203, -43.1335) radius 1.6 construction
  arc A51 (-21.4111, -8.4003) -> (-24.6871, -7.7166) centre (-23.2729, -9.1308) ccw construction
  arc A52 (-21.4111, -8.4003) -> (-8.4003, -21.4111) centre (0, 0) ccw construction
  arc A53 (-7.7166, -24.6871) -> (-8.4003, -21.4111) centre (-9.1308, -23.2729) ccw construction
  line L51 (-7.7166, -24.6871) -> (-20.8597, -37.8302) construction
  arc A54 (-23.6881, -37.8302) -> (-20.8597, -37.8302) centre (-22.2739, -36.416) ccw construction
  line L52 (-23.6881, -37.8302) -> (-37.8302, -23.6881) construction
  arc A55 (-37.8302, -20.8597) -> (-37.8302, -23.6881) centre (-36.416, -22.2739) ccw construction
  line L53 (-37.8302, -20.8597) -> (-24.6871, -7.7166) construction
  circle A56 centre (-43.1335, -21.9203) radius 1.6 construction
  circle A57 centre (43.1335, 21.9203) radius 1.6 construction
  circle A58 centre (21.9203, 43.1335) radius 1.6 construction
  circle A59 centre (-21.9203, -43.1335) radius 1.6 construction
  circle A60 centre (-43.1335, 21.9203) radius 1.6 construction
  circle A61 centre (0, 0) radius 18 construction
  circle A62 centre (43.1335, -21.9203) radius 1.6 construction
  circle A63 centre (0, 22) radius 1.6 construction
  circle A64 centre (-22, 0) radius 1.6 construction
  circle A65 centre (0, -22) radius 1.6 construction
  circle A66 centre (22, 0) radius 1.6 construction
  arc A67 (-46.3155, -85.2064) -> (-46.3155, -73.8927) centre (-51.9723, -79.5495) ccw construction
  line L54 (-46.3155, -85.2064) -> (-49.3795, -88.2704) construction
  arc A68 (-49.3795, -88.2704) -> (-48.6481, -93.0503) centre (-47.2582, -90.3917) ccw construction
  arc A69 (-48.6481, -93.0503) -> (-45.42, -94.668) centre (0, 0) ccw construction
  arc A70 (-45.42, -94.668) -> (-43.0355, -94.1655) centre (-44.5548, -92.8648) ccw construction
  line L55 (-43.0355, -94.1655) -> (-18.3802, -65.3664) construction
  arc A71 (-17.477, -64.7643) -> (-18.3802, -65.3664) centre (-16.8609, -66.6671) ccw construction
  line L56 (-17.477, -64.7643) -> (-0.6161, -59.3045) construction
  arc A72 (0.6161, -59.3045) -> (-0.6161, -59.3045) centre (0, -61.2072) ccw construction
  line L57 (0.6161, -59.3045) -> (17.477, -64.7643) construction
  arc A73 (18.3802, -65.3664) -> (17.477, -64.7643) centre (16.8609, -66.6671) ccw construction
  line L58 (18.3802, -65.3664) -> (43.0355, -94.1655) construction
  arc A74 (43.0355, -94.1655) -> (45.42, -94.668) centre (44.5548, -92.8648) ccw construction
  arc A75 (45.42, -94.668) -> (48.6481, -93.0503) centre (0, 0) ccw construction
  arc A76 (48.6481, -93.0503) -> (49.3795, -88.2704) centre (47.2582, -90.3917) ccw construction
  line L59 (49.3795, -88.2704) -> (46.3155, -85.2064) construction
  arc A77 (46.3155, -73.8927) -> (46.3155, -85.2064) centre (51.9723, -79.5495) ccw construction
  line L60 (46.3155, -73.8927) -> (73.8927, -46.3155) construction
  arc A78 (85.2064, -46.3155) -> (73.8927, -46.3155) centre (79.5495, -51.9723) ccw construction
  line L61 (85.2064, -46.3155) -> (88.2704, -49.3795) construction
  arc A79 (88.2704, -49.3795) -> (93.0503, -48.6481) centre (90.3917, -47.2582) ccw construction
  arc A80 (93.0503, -48.6481) -> (93.0503, 48.6481) centre (0, 0) ccw construction
  arc A81 (93.0503, 48.6481) -> (88.2704, 49.3795) centre (90.3917, 47.2582) ccw construction
  line L62 (88.2704, 49.3795) -> (85.2064, 46.3155) construction
  arc A82 (73.8927, 46.3155) -> (85.2064, 46.3155) centre (79.5495, 51.9723) ccw construction
  line L63 (73.8927, 46.3155) -> (46.3155, 73.8927) construction
  arc A83 (46.3155, 85.2064) -> (46.3155, 73.8927) centre (51.9723, 79.5495) ccw construction
  line L64 (46.3155, 85.2064) -> (49.3795, 88.2704) construction
  arc A84 (49.3795, 88.2704) -> (48.6481, 93.0503) centre (47.2582, 90.3917) ccw construction
  arc A85 (48.6481, 93.0503) -> (-48.6481, 93.0503) centre (0, 0) ccw construction
  arc A86 (-48.6481, 93.0503) -> (-49.3795, 88.2704) centre (-47.2582, 90.3917) ccw construction
  line L65 (-49.3795, 88.2704) -> (-46.3155, 85.2064) construction
  arc A87 (-46.3155, 73.8927) -> (-46.3155, 85.2064) centre (-51.9723, 79.5495) ccw construction
  line L66 (-46.3155, 73.8927) -> (-73.8927, 46.3155) construction
  arc A88 (-85.2064, 46.3155) -> (-73.8927, 46.3155) centre (-79.5495, 51.9723) ccw construction
  line L67 (-85.2064, 46.3155) -> (-88.2704, 49.3795) construction
  arc A89 (-88.2704, 49.3795) -> (-93.0503, 48.6481) centre (-90.3917, 47.2582) ccw construction
  arc A90 (-93.0503, 48.6481) -> (-93.0503, -48.6481) centre (0, 0) ccw construction
  arc A91 (-93.0503, -48.6481) -> (-88.2704, -49.3795) centre (-90.3917, -47.2582) ccw construction
  line L68 (-88.2704, -49.3795) -> (-85.2064, -46.3155) construction
  arc A92 (-73.8927, -46.3155) -> (-85.2064, -46.3155) centre (-79.5495, -51.9723) ccw construction
  line L69 (-73.8927, -46.3155) -> (-46.3155, -73.8927) construction
  circle A93 centre (-37.8302, 79.5495) radius 1.6 construction
  circle A94 centre (-79.5495, 37.8302) radius 1.6 construction
  circle A95 centre (-79.5495, -37.8302) radius 1.6 construction
  circle A96 centre (79.5495, -37.8302) radius 1.6 construction
  circle A97 centre (37.8302, 79.5495) radius 1.6 construction
  circle A98 centre (79.5495, 37.8302) radius 1.6 construction
  circle A99 centre (-20.5578, -60.8546) radius 1.55 construction
  circle A100 centre (20.5578, -60.8546) radius 1.55 construction
  circle A101 centre (37.8302, -79.5495) radius 1.6 construction
  circle A102 centre (-37.8302, -79.5495) radius 1.6 construction
  line L70 (-46.669, 63.6396) -> (-27.2236, 44.1942) construction
  arc A103 (-27.2236, 41.3657) -> (-27.2236, 44.1942) centre (-28.6378, 42.78) ccw construction
  line L71 (-27.2236, 41.3657) -> (-41.3657, 27.2236) construction
  arc A104 (-44.1942, 27.2236) -> (-41.3657, 27.2236) centre (-42.78, 28.6378) ccw construction
  line L72 (-44.1942, 27.2236) -> (-63.6396, 46.669) construction
  line L73 (-63.6396, 46.669) -> (-46.669, 63.6396) construction
  line L74 (8.5, 90.5) -> (8.5, 101.3496)
  line L75 (0, 0) -> (0, 105) construction
  arc A105 (48.6481, 93.0503) -> (-48.6481, 93.0503) centre (0, 0) ccw construction
  line L76 (-8.5, 90.5) -> (-8.5, 101.3496)
  arc A106 (48.6481, 93.0503) -> (-48.6481, 93.0503) centre (0, 0) ccw construction
  line L77 (7, 89) -> (-7, 89)
  line L78 (11.5, 84) -> (-11.5, 84)
  line L79 (14.5, 87) -> (14.5, 93.3742)
  arc A107 (37.7453, 90.4395) -> (-37.7453, 90.4395) centre (0, 0) ccw construction
  arc A108 (37.7453, 90.4395) -> (-37.7453, 90.4395) centre (0, 0) ccw construction
  arc A109 (37.7453, 90.4395) -> (18.0526, 96.3229) centre (0, 0) ccw construction
  arc A110 (-48.6481, 93.0503) -> (-49.3795, 88.2704) centre (-47.2582, 90.3917) ccw construction
  arc A111 (48.6481, 93.0503) -> (11.8382, 104.3305) centre (0, 0) ccw construction
  arc A112 (14.5, 96.9214) -> (-37.7453, 90.4395) centre (0, 0) ccw construction
  arc A113 (18.0526, 96.3229) -> (14.5, 93.3742) centre (17.5, 93.3742) ccw
  arc A114 (-14.5, 93.3742) -> (-18.0526, 96.3229) centre (-17.5, 93.3742) ccw
  arc A115 (-8.5, 90.5) -> (-7, 89) centre (-7, 90.5) ccw
  line L80 (18.0526, 96.3229) -> (18.0526, 103.4365)
  line L81 (-18.0526, 96.3229) -> (-18.0526, 103.4365)
  arc A116 (18.0526, 103.4365) -> (-18.0526, 103.4365) centre (0, 0) ccw
  arc A117 (-11.8382, 104.3305) -> (-48.6481, 93.0503) centre (0, 0) ccw construction
  arc A118 (11.8382, 104.3305) -> (8.5, 101.3496) centre (11.5, 101.3496) ccw
  arc A119 (-8.5, 101.3496) -> (-11.8382, 104.3305) centre (-11.5, 101.3496) ccw
  arc A120 (7, 89) -> (8.5, 90.5) centre (7, 90.5) ccw
  arc A121 (11.5, 84) -> (14.5, 87) centre (11.5, 87) ccw
  line L82 (-14.5, 87) -> (-14.5, 93.3742)
  arc A122 (-14.5, 87) -> (-11.5, 84) centre (-11.5, 87) ccw
  arc A123 (47.1257, -21.6698) -> (43.384, -17.9282) centre (43.1335, -21.9203) ccw projected
  line L83 (43.384, -17.9282) -> (26.8701, -1.4142) projected
  arc A124 (43.384, 17.9282) -> (47.1257, 21.6698) centre (43.1335, 21.9203) ccw projected
  line L84 (47.1257, 21.6698) -> (67.8823, 42.4264) projected
  arc A125 (21.6698, 47.1257) -> (17.9282, 43.384) centre (21.9203, 43.1335) ccw projected
  line L85 (17.9282, 43.384) -> (1.4142, 26.8701) projected
  arc A126 (-17.9282, 43.384) -> (-21.6698, 47.1257) centre (-21.9203, 43.1335) ccw projected
  line L86 (-21.6698, 47.1257) -> (-42.4264, 67.8823) projected
  line L87 (-67.8823, 42.4264) -> (-47.1257, 21.6698) projected
  arc A127 (-47.1257, 21.6698) -> (-43.384, 17.9282) centre (-43.1335, 21.9203) ccw projected
  line L88 (-26.8701, -1.4142) -> (-43.384, -17.9282) projected
  arc A128 (-43.384, -17.9282) -> (-47.1257, -21.6698) centre (-43.1335, -21.9203) ccw projected
  line L89 (-42.4264, -67.8823) -> (-21.6698, -47.1257) projected
  arc A129 (-21.6698, -47.1257) -> (-17.9282, -43.384) centre (-21.9203, -43.1335) ccw projected
  line L90 (1.4142, -26.8701) -> (17.9282, -43.384) projected
  arc A130 (17.9282, -43.384) -> (21.6698, -47.1257) centre (21.9203, -43.1335) ccw projected
  point P0 (8.5, 89)
  point P1 (8.5, 104.6554)
  point P2 (-8.5, 89)
  point P3 (-8.5, 104.6554)
  point P4 (14.5, 84)
  point P5 (-14.5, 84)
  point P6 (14.5, 84)
  point P7 (14.5, 84)
  dimension "d83" = 17
  dimension "d85" = 5
  dimension "d86" = 21
  dimension "d87" = 6
  dimension "d88" = 3
  dimension "d90" = 3
  dimension "d95" = 1.5
  dimension "d96" = 3
  constraints: 40 point on circle, 18 end point, 13 centre point, 12 point on line, 11 tangent, 10 symmetric about line, 4 vertical, 2 equal radius, 2 parallel, 1 coincident, 1 perpendicular, 3 other
  measures "d83" distance between parallel lines of L74 L76
  measures "d85" distance between parallel lines of L77 L78
  measures "d86" distance from line of L78 L75.end
  measures "d87" distance between parallel lines of L74 L79
  measures "d88" radius of A113
  measures "d90" radius of A118
  measures "d95" radius of A115
  measures "d96" radius of A121
extrude "Выдавливание3" cut sketch "Эскиз3" along normal mid plane 22 contours A120 L77 A115 L76 A119 A116 A118 L74
extrude "Выдавливание4" add sketch "Эскиз3" against normal blind 2 contours L74 A118 A116 L80 A113 L79 A121 L78 A122 L82 A114 L81 A119 L76 A115 L77 A120